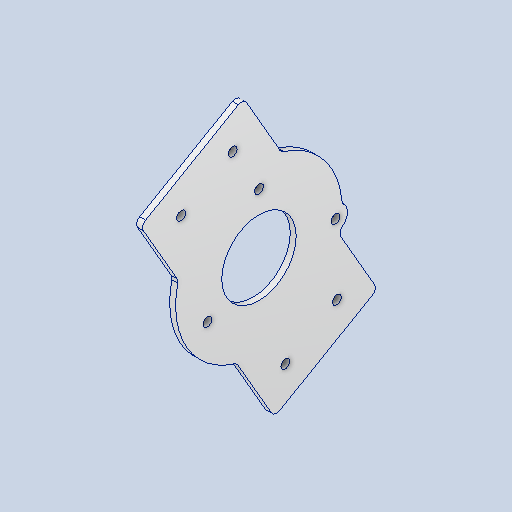
# Autodesk Inventor part: hand-grab-v3-Plate-ASP_F
Saved by Autodesk Inventor 2025.2 (Build 292293000, 293)
## iProperties
Created: 2024-11-30
Part Number: hand-grab-v3-Plate-ASP_F
Material: アルミニウム 6061
Document SubType Name: Modeling
Designer: haruy
Density: 2.7 g/cm^3
Appearance: アルミニウム - フラット
Author: haruy
Autodesk Inventor part; units mm, degrees
ref_plane "YZ Plane" through (0, 0, 0) normal (1, 0, 0) x (0, 1, 0)
ref_plane "XZ Plane" through (0, 0, 0) normal (0, 1, 0) x (-1, 0, 0)
ref_plane "XY Plane" through (0, 0, 0) normal (0, 0, 1) x (1, 0, 0)
sketch "スケッチ5" plane through (0, 0, 0) normal (1, 0, 0) x (0, 1, 0)
  circle A0 centre (68.5779, -0.3457) radius 120
  line L0 (68.5779, -0.3457) -> (-262.8846, -0.3457) construction
  line L1 (136.0779, -117.2592) -> (-66.4221, -0.3457)
  circle A1 centre (68.5779, -0.3457) radius 5
  line L2 (68.5779, -0.3457) -> (136.0779, 116.5677) construction
  line L3 (68.5779, -0.3457) -> (136.0779, -117.2592) construction
  line L4 (68.5779, -0.3457) -> (-66.4221, -0.3457)
  line L5 (85.6138, 37.1613) -> (80.6138, 28.5011) construction
  line L6 (80.6138, 28.5011) -> (84.0779, 26.5011) construction
  line L7 (84.0779, 26.5011) -> (89.0779, 35.1613) construction
  line L8 (89.0779, 35.1613) -> (85.6138, 37.1613)
  line L9 (89.0779, 35.1613) -> (84.0779, 26.5011) construction
  line L10 (84.0779, 26.5011) -> (87.542, 24.5011) construction
  line L11 (87.542, 24.5011) -> (92.542, 33.1613) construction
  line L12 (92.542, 33.1613) -> (89.0779, 35.1613)
  line L13 (83.1138, 32.8312) -> (90.042, 28.8312) construction
  circle A2 centre (68.5779, -0.3457) radius 2.65 construction
  line L14 (85.3973, 37.2863) -> (78.8973, 26.028) construction
  line L15 (78.8973, 26.028) -> (74.5672, 28.528) construction
  line L16 (74.5672, 28.528) -> (81.0672, 39.7863) construction
  line L17 (81.0672, 39.7863) -> (85.3973, 37.2863)
  line L18 (92.7585, 33.0363) -> (86.2585, 21.778) construction
  line L19 (86.2585, 21.778) -> (90.5886, 19.278) construction
  line L20 (90.5886, 19.278) -> (97.0886, 30.5363) construction
  line L21 (97.0886, 30.5363) -> (92.7585, 33.0363)
  circle A3 centre (68.5779, -0.3457) radius 28.3207 construction
  line L22 (27.5779, 8.9043) -> (27.5779, 3.9043)
  line L23 (27.5779, 3.9043) -> (40.5779, 3.9043) construction
  line L24 (40.5779, 8.9043) -> (27.5779, 8.9043) construction
  line L25 (40.5779, 3.9043) -> (40.5779, 8.9043)
  line L26 (27.5779, -4.5957) -> (40.5779, -4.5957) construction
  line L27 (27.5779, -9.5957) -> (27.5779, -4.5957)
  line L28 (40.5779, -9.5957) -> (27.5779, -9.5957) construction
  line L29 (40.5779, -4.5957) -> (40.5779, -9.5957)
  line L30 (81.0672, -40.4778) -> (85.3973, -37.9778)
  line L31 (85.3973, -37.9778) -> (78.8973, -26.7194) construction
  line L32 (74.5672, -29.2194) -> (81.0672, -40.4778) construction
  line L33 (78.8973, -26.7194) -> (74.5672, -29.2194) construction
  line L34 (92.7585, -33.7278) -> (86.2585, -22.4694) construction
  line L35 (97.0886, -31.2278) -> (92.7585, -33.7278)
  line L36 (90.5886, -19.9694) -> (97.0886, -31.2278) construction
  line L37 (86.2585, -22.4694) -> (90.5886, -19.9694) construction
  line L38 (74.5672, 28.528) -> (73.9509, 27.4606)
  line L39 (90.5886, 19.278) -> (89.9724, 18.2106) construction
  line L40 (40.5779, 8.9043) -> (41.8104, 8.9043)
  line L41 (40.5779, -9.5957) -> (41.8104, -9.5957)
  line L42 (74.5672, -29.2194) -> (70.7713, -22.6449)
  line L43 (90.5886, -19.9694) -> (89.9724, -18.9021) construction
  line L44 (82.1888, 31.229) -> (72.1888, 13.9085) construction
  line L45 (72.1888, 13.9085) -> (66.9926, 16.9085) construction
  line L46 (66.9926, 16.9085) -> (76.9926, 34.229) construction
  line L47 (76.9926, 34.229) -> (82.1888, 31.229)
  circle A4 centre (72.0907, 19.7387) radius 1.5
  circle A5 centre (77.0907, 28.3989) radius 1.5
  circle A6 centre (84.2151, 12.7387) radius 1.5
  circle A7 centre (89.2151, 21.3989) radius 1.5
  circle A8 centre (39.4279, 6.6543) radius 1.5
  circle A9 centre (49.4279, 6.6543) radius 1.5
  circle A10 centre (49.4279, -7.3457) radius 1.5
  circle A11 centre (39.4279, -7.3457) radius 1.5
  circle A12 centre (77.0907, -29.0904) radius 1.5
  circle A13 centre (72.0907, -20.4301) radius 1.5
  circle A14 centre (84.2151, -13.4301) radius 1.5
  circle A15 centre (89.2151, -22.0904) radius 1.5
  line L48 (69.5907, 15.4085) -> (82.1888, 31.229) construction
  circle A16 centre (68.5779, -0.3457) radius 34.3835
  line L49 (60.5779, 46.6543) -> (-119.4221, 46.6543) construction
  line L50 (-119.4221, 46.6543) -> (-119.4221, 31.6543)
  line L51 (-119.4221, 31.6543) -> (60.5779, 31.6543) construction
  line L52 (60.5779, 31.6543) -> (60.5779, 46.6543) construction
  circle A17 centre (50.5779, 39.1543) radius 1.5 construction
  circle A18 centre (40.5779, 39.1543) radius 1.5 construction
  line L53 (34.1944, 46.6543) -> (34.1944, -0.3457) construction
  line L54 (60.5779, 46.6543) -> (87.898, 28.0965) construction
  line L55 (34.1944, -47.3457) -> (34.1944, -0.3457) construction
  line L56 (60.5779, -47.3457) -> (87.898, -28.7879) construction
  line L57 (60.5779, -47.3457) -> (-119.4221, -47.3457) construction
  line L58 (-119.4221, -32.3457) -> (60.5779, -32.3457) construction
  circle A19 centre (40.5779, -39.8457) radius 1.5 construction
  circle A20 centre (50.5779, -39.8457) radius 1.5 construction
  line L59 (68.5779, -0.3457) -> (51.3862, 29.4312)
  line L60 (53.2382, 46.2235) -> (35.9176, 36.2235)
  line L61 (35.9176, 36.2235) -> (40.9176, 27.5632)
  line L62 (40.9176, 27.5632) -> (58.2382, 37.5632)
  line L63 (58.2382, 37.5632) -> (53.2382, 46.2235)
  circle A21 centre (51.408, 39.3934) radius 1.5
  circle A22 centre (42.7478, 34.3934) radius 1.5
  circle A23 centre (42.7478, -35.0848) radius 1.5
  circle A24 centre (51.408, -40.0848) radius 1.5
  circle A25 centre (111.5779, -5.3457) radius 1.5
  circle A26 centre (111.5779, 4.6543) radius 1.5
  circle A27 centre (68.5779, -0.3457) radius 193.5
  line L64 (-124.2868, 15.3208) -> (151.4426, 174.5133)
  line L65 (68.5779, -0.3457) -> (8.5779, 103.5773)
  line L66 (68.5779, -0.3457) -> (68.5779, 193.1543)
  line L67 (117.549, 4.8338) -> (16.049, 180.6369)
  line L68 (16.049, 180.6369) -> (-1.2715, 170.6369)
  line L69 (-1.2715, 170.6369) -> (100.2285, -5.1662)
  line L70 (100.2285, -5.1662) -> (117.549, 4.8338)
  circle A28 centre (37.9737, 117.6622) radius 1.5
  circle A29 centre (13.3039, 170.3917) radius 1.5
  circle A30 centre (58.5779, 16.9748) radius 1.5
  circle A31 centre (68.5779, -0.3457) radius 10 construction
  circle A32 centre (103.8888, 8.494) radius 1.5
  circle A33 centre (93.8888, 25.8145) radius 1.5
  line L71 (117.549, 4.8338) -> (90.6574, -10.6921)
  line L72 (97.549, 39.4748) -> (64.1622, 20.1989)
  line L73 (19.6068, -5.5252) -> (52.9936, 13.7507)
  circle A34 centre (33.267, -9.1855) radius 1.5
  circle A35 centre (43.267, -26.506) radius 1.5
  line L74 (39.6068, -40.1662) -> (-61.8932, 135.6369)
  line L75 (56.9273, -30.1662) -> (39.6068, -40.1662)
  line L76 (39.6068, -40.1662) -> (66.4984, -24.6404)
  line L77 (68.5779, -0.3457) -> (51.3862, -30.1227)
  line L78 (69.2071, -12.256) -> (57.9487, -5.756) construction
  line L79 (57.9487, -5.756) -> (48.9487, -21.3444) construction
  line L80 (48.9487, -21.3444) -> (60.2071, -27.8444) construction
  line L81 (60.2071, -27.8444) -> (69.2071, -12.256) construction
  circle A36 centre (68.5779, -0.3457) radius 28
  circle A37 centre (68.5779, -0.3457) radius 38 construction
  circle A38 centre (68.5779, -0.3457) radius 12.5
  circle A39 centre (58.5779, -17.6662) radius 1.5
  circle A40 centre (88.5779, -0.3457) radius 1.5
  circle A41 centre (66.9902, -26.0957) radius 4
  circle A42 centre (66.9902, -26.0957) radius 1.5
  line L82 (58.2382, 37.5632) -> (60.7896, 33.144)
  line L83 (40.9176, 27.5632) -> (43.4691, 23.144)
  line L84 (58.2382, -38.2547) -> (60.7896, -33.8355)
  line L85 (53.2382, -46.915) -> (58.2382, -38.2547)
  line L86 (35.9176, -36.915) -> (53.2382, -46.915)
  circle A43 centre (51.408, -40.0848) radius 1.5
  circle A44 centre (42.7478, -35.0848) radius 1.5
  line L87 (40.9176, -28.2547) -> (35.9176, -36.915)
  line L88 (40.9176, -28.2547) -> (43.4691, -23.8355)
  line L89 (106.5779, 9.6543) -> (101.4751, 9.6543)
  line L90 (116.5779, 9.6543) -> (106.5779, 9.6543)
  line L91 (116.5779, -10.3457) -> (116.5779, 9.6543)
  circle A45 centre (111.5779, 4.6543) radius 1.5
  circle A46 centre (111.5779, -5.3457) radius 1.5
  line L92 (106.5779, -10.3457) -> (116.5779, -10.3457)
  line L93 (106.5779, -10.3457) -> (101.4751, -10.3457)
  point P0 (0, 0)
  point P1 (53.4487, -13.5502)
  point P2 (44.5779, 41.2235)
  point P3 (44.5779, -41.915)
  point P4 (116.5779, -0.3457)
  point P5 (41.6073, 7.1768)
  point P6 (61.6073, -27.4642)
  point P7 (63.4018, -27.8632)
  point P8 (70.3342, -28.2906)
  point P9 (95.5485, -7.8683)
  point P10 (100.2285, -5.1662)
  point P11 (75.5485, 26.7727)
  dimension "d169" = 3
  dimension "d170" = 3
  dimension "d171" = 10
  dimension "d172" = 10
  dimension "d173" = 7.5
  dimension "d174" = 7.5
  dimension "d175" = 60
  dimension "d176" = 10
  dimension "d177" = 10
  dimension "d178" = 10
  dimension "d179" = 3
  dimension "d180" = 5
  dimension "d181" = 5
  dimension "d182" = 360
  dimension "d183" = 387
  dimension "d184" = 110
  dimension "d185" = 60
  dimension "d186" = 20
  dimension "d187" = 73
  dimension "d188" = 3
  dimension "d189" = 3
  dimension "d190" = 7.5
  dimension "d191" = 7.5
  dimension "d192" = 7.5
  dimension "d193" = 7.5
  dimension "d194" = 3
  dimension "d195" = 20
  dimension "d196" = 20
  dimension "d197" = 3
  dimension "d198" = 3
  dimension "d199" = 10
  dimension "d200" = 10
  dimension "d201" = 10
  dimension "d202" = 20
  dimension "d203" = 10
  dimension "d204" = 120
  dimension "d205" = 13
  dimension "d206" = 18
  dimension "d207" = 6.5
  dimension "d208" = 56
  dimension "d209" = 10
  dimension "d210" = 25
  dimension "d211" = 25
  dimension "d212" = 20
  dimension "d213" = 360
  dimension "d214" = 8
  dimension "d215" = 5
  dimension "d216" = 5
  dimension "d217" = 3
  dimension "d218" = 360
  constraints: 188 end point, 45 centre point, 17 symmetric about line, 9 point on line, 8 parallel, 6 coincident, 6 perpendicular, 4 midpoint, 3 point on circle, 2 collinear, 2 tangent, 1 vertical, 86 other
  measures "d169" diameter of A17
  measures "d170" diameter of A18
  measures "d171" distance from line of A17.centre L52
  measures "d172" distance of A18.centre A17.centre
  measures "d173" distance from line of A17.centre L49
  measures "d174" distance from line of L49 A18.centre
  measures "d176" distance between parallel lines of L60 L62
  measures "d177" distance between parallel lines of L63 L59
  measures "d178" distance between parallel lines of L59 L61
  measures "d179" diameter of A21
  measures "d180" distance from line of L59 A21.centre
  measures "d181" distance from line of A21.centre L60
  measures "d183" diameter of A27
  measures "d184" distance from line of L64 A3.centre
  measures "d186" distance of L68.end L67.end
  measures "d187" distance between parallel lines of L64 L68
  measures "d188" diameter of A28
  measures "d189" diameter of A29
  measures "d190" distance from line of A28.centre L64
  measures "d191" distance from line of A28.centre L69
  measures "d192" distance from line of A29.centre L68
  measures "d193" distance from line of A29.centre L67
  measures "d194" diameter of A30
  measures "d195" diameter of A31
  measures "d196" distance from line of L70 point (68.578, -0.346)
  measures "d197" diameter of A32
  measures "d198" diameter of A33
  measures "d199" distance from line of A32.centre L70
  measures "d200" distance from line of L67 A33.centre
  measures "d201" distance from line of L67 A32.centre
  measures "d202" distance of A33.centre A32.centre
  measures "d203" distance from line of L72 A33.centre
  measures "d205" distance from line of point (53.449, -13.55) L81
  measures "d206" distance between parallel lines of L78 L80
  measures "d207" distance between parallel lines of L77 L81
  measures "d208" diameter of A36
  measures "d209" radial gap between concentric circles of A36 A37
  measures "d210" diameter of A38
  measures "d211" distance from line of L69 L4.start
  measures "d212" distance of point (68.578, -0.346) A30.centre
  measures "d214" diameter of A41
  measures "d215" distance from line of L81 A41.centre
  measures "d216" distance from line of A41.centre L42
  measures "d217" diameter of A42
extrude "押し出し4" add sketch "スケッチ5" against normal blind 2 contours L67 L90 L89 A32 A16 L72 | L67 L91 L70 A16 L89 A32 L90 | A36 L72 L66 | L66 A38 L59 A30 A36 | L67 L70 L91 | A16 L70 L69 A36 L72 | L73 A16 L4 | L4 A16 L88 A35 L87 L74 L73 | L69 A36 L72 A5 | L72 A36 L69 A41 L76 L77 A39 A38 L66 | L59 A30 A38 L4 A36 | A16 L73 A8 A36 L4 | L4 A36 L77 A16 | L87 L88 A35 A16 L75 L86 L74 | A36 L69 | A5 L72 | A38 L77 A1 L66 | L66 A1 L59 A38 | L4 A38 L77 A39 A36 | L73 L25 A8 | L86 L75 L74 | L69 L71 A36 | L59 A1 L4 A38 | A8 L25 L73 | L4 A1 L77 A38 | A36 L76 L75 A16 L77 | A39 L77 | L77 A39 | L76 A41 A36 | A41 A36 | A36 A41 | A11 L29 | L29 A11 | A4 | A6 | A7 | A9 | A10 | A13 | A14 | A23 | A26 picked at (77.6802, 27.4001) picked at (39.3486, 5.7524) picked at (40.6415, 6.0852)
extrude "押し出し5" cut sketch "スケッチ5" against normal blind 2 contours A38 L77 A1 L66 | L66 A1 L59 A38 | L59 A1 L4 A38 | L4 A1 L77 A38
fillet "フィレット4" radius 2 10 edges at (-1, 95.5485, -7.8683) (-1, 117.549, 4.8338) (-1, 97.549, 39.4748) (-1, 75.5485, 26.7727) (-1, 41.6073, 7.1768) (-1, 19.6068, -5.5252) (-1, 39.6068, -40.1662) (-1, 61.6073, -27.4642) (-1, 63.4018, -27.8632) (-1, 70.3342, -28.2906)
equation "\"d174\" = d173"
equation "\"d200\" = d201"
